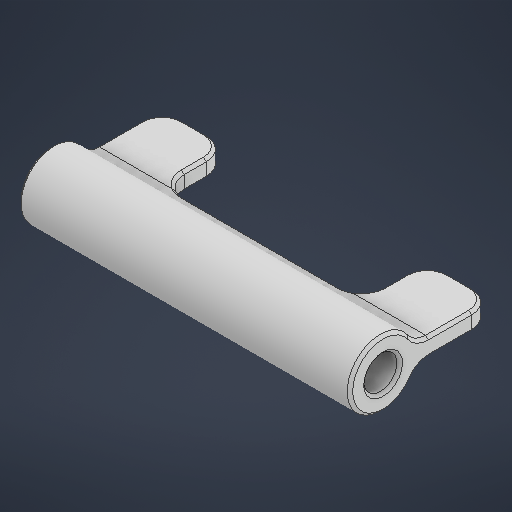
# Autodesk Inventor part: CoinLockUpperRow
Saved by Autodesk Inventor 2026.3 (Build 303398000, 398)
## iProperties
Created: 2026-05-05
Part Number: CoinLockUpperRow
Material: Generic
Document SubType Name: Modeling
Designer: frede
Density: 1 g/cm^3
Appearance: Default
Author: frede
Autodesk Inventor part; units mm, degrees
ref_plane "YZ Plane" through (0, 0, 0) normal (1, 0, 0) x (0, 1, 0)
ref_plane "XZ Plane" through (0, 0, 0) normal (0, 1, 0) x (-1, 0, 0)
ref_plane "XY Plane" through (0, 0, 0) normal (0, 0, 1) x (1, 0, 0)
sketch "Sketch3" plane through (0, 0, 0) normal (1, 0, 0) x (0, 1, 0)
  circle A0 centre (0, 0) radius 1.5
  arc A1 (1.725, -2.4545) -> (-1.6531, -2.5034) centre (0, 0) ccw
  line L0 (-0.7552, -4.1724) -> (-0.7552, -10)
  line L1 (-0.7552, -10) -> (0.875, -10)
  line L2 (0.875, -10) -> (0.875, -4.0908)
  arc A2 (1.725, -2.4545) -> (0.875, -4.0908) centre (2.875, -4.0908) ccw
  arc A3 (-0.7552, -4.1724) -> (-1.6531, -2.5034) centre (-2.7552, -4.1724) ccw
  dimension "d4" = 3
  dimension "d5" = 6
  dimension "d7" = 2
  constraints: 6 end point, 6 point on circle, 4 centre point, 4 tangent, 2 coincident, 1 equal radius, 1 parallel
  measures "d4" diameter of A0
  measures "d5" diameter of A1
  measures "d7" radius of A2
extrude "Extrusion2" add sketch "Sketch3" along normal blind 30
sketch "Sketch5" plane through (0, 0.875, -4.0908) normal (0, 1, 0) x (1, 0, 0)
  line L0 (0, 5.9092) -> (30, 5.9092) projected
  line L1 (6, 5.9092) -> (24, 5.9092)
  line L2 (24, 5.9092) -> (24, -0.0908)
  line L3 (24, -0.0908) -> (6, -0.0908)
  line L4 (6, -0.0908) -> (6, 5.9092)
  line L5 (0, 5.9092) -> (0, 0) projected
  point P0 (0, -4.0908)
  dimension "d18" = 6
  dimension "d19" = 30
  dimension "d20" = 6
  dimension "d21" = 18
  constraints: 8 end point, 2 parallel, 1 horizontal, 1 perpendicular, 1 point on line
  measures "d18" distance of L1.end L2.end
  measures "d19" distance of L0.start L0.end
  measures "d20" distance between parallel lines of L5 L4
  measures "d21" distance between parallel lines of L2 L4
extrude "Extrusion3" cut sketch "Sketch5" along normal blind 0.5 and the other way blind 2
fillet "Fillet1" radius 2 6 edges at (6, 0.0599, -10) (24, 0.0599, -10) (30, 0.0599, -10) (0, 0.0599, -10) (24, 0.0572, -4) (6, 0.0572, -4)
chamfer "Chamfer2" distance 0.25 angle 45 38 edges at (5.4142, 0.875, -9.4142) (6, 0.875, -7) (6.3889, 0.875, -4.815) (7.6998, 0.8762, -4.0227) (15, 0.8771, -4) (22.3002, 0.8762, -4.0227) (23.6111, 0.875, -4.815) (24, 0.875, -7) (24.5858, 0.875, -9.4142) (27, 0.875, -10) (29.4142, 0.875, -9.4142) (30, 0.875, -6.0454) (30, 1.1002, -3.1688) (30, -0.0435, 2.9997) (30, -0.9939, -3.2248) (30, -0.7552, -6.0862) (29.4142, -0.7552, -9.4142) (27, -0.7552, -10) (24.5858, -0.7552, -9.4142) (24, -0.7552, -7) (23.677, -0.7552, -4.9102) (22.4123, -0.7594, -4.043) (15, -0.7626, -4) (7.5877, -0.7594, -4.043) (6.323, -0.7552, -4.9102) (6, -0.7552, -7) (5.4142, -0.7552, -9.4142) (3, -0.7552, -10) (0.5858, -0.7552, -9.4142) (0, -0.7552, -6.0862) (0, -0.9939, -3.2248) (0, -0.0435, 2.9997) (0, 1.1002, -3.1688) (0, 0.875, -6.0454) (0.5858, 0.875, -9.4142) (3, 0.875, -10) (30, -1.5, 0) (0, -1.5, 0)
equation "\"d20\" = -0.5 * d21 + 0.5 * d19"
body "Solid2"
